Autodesk Fusion 360 part; units mm, degrees
note: some values were not read from the file. Set by a fixed rule: which sketch regions a step uses.
(part 2 of 2)
component "Component'''''''''''''" placed x (1, 0, 0) y (0, 1, 0) z (0, 0, 1) at (0, 0, 0)
component "Component''''''''''''''" placed x (1, 0, 0) y (0, 1, 0) z (0, 0, 1) at (0, 0, 0)
component "Component'''''''''''''''" placed x (1, 0, 0) y (0, 1, 0) z (0, 0, 1) at (0, 0, 0)
component "Component''''''''''''''''" placed x (1, 0, 0) y (0, 1, 0) z (0, 0, 1) at (0, 0, 0)
component "Component'''''''''''''''''" placed x (1, 0, 0) y (0, 1, 0) z (0, 0, 1) at (0, 0, 0)
component "Component''''''''''''''''''" placed x (1, 0, 0) y (0, 1, 0) z (0, 0, 1) at (0, 0, 0)
component "Component'''''''''''''''''''" placed x (1, 0, 0) y (0, 1, 0) z (0, 0, 1) at (0, 0, 0)
component "Component''''''''''''''''''''" placed x (1, 0, 0) y (0, 1, 0) z (0, 0, 1) at (0, 0, 0)
component "Component'''''''''''''''''''''" placed x (1, 0, 0) y (0, 1, 0) z (0, 0, 1) at (0, 0, 0)
component "Component''''''''''''''''''''''" placed x (1, 0, 0) y (0, 1, 0) z (0, 0, 1) at (0, 0, 0)
component "Component'''''''''''''''''''''''" placed x (1, 0, 0) y (0, 1, 0) z (0, 0, 1) at (0, 0, 0)
component "Component''''''''''''''''''''''''" placed x (1, 0, 0) y (0, 1, 0) z (0, 0, 1) at (0, 0, 0)
component "Component'''''''''''''''''''''''''" placed x (1, 0, 0) y (0, 1, 0) z (0, 0, 1) at (0, 0, 0)
component "Component''''''''''''''''''''''''''" placed x (1, 0, 0) y (0, 1, 0) z (0, 0, 1) at (0, 0, 0)
component "Component'''''''''''''''''''''''''''" placed x (1, 0, 0) y (0, 1, 0) z (0, 0, 1) at (0, 0, 0)
component "Component''''''''''''''''''''''''''''" placed x (1, 0, 0) y (0, 1, 0) z (0, 0, 1) at (0, 0, 0)
component "Component'''''''''''''''''''''''''''''" placed x (1, 0, 0) y (0, 1, 0) z (0, 0, 1) at (0, 0, 0)
component "Component''''''''''''''''''''''''''''''" placed x (1, 0, 0) y (0, 1, 0) z (0, 0, 1) at (0, 0, 0)
component "Component'''''''''''''''''''''''''''''''" placed x (1, 0, 0) y (0, 1, 0) z (0, 0, 1) at (0, 0, 0)
component "Component''''''''''''''''''''''''''''''''" placed x (1, 0, 0) y (0, 1, 0) z (0, 0, 1) at (0, 0, 0)
component "Component'''''''''''''''''''''''''''''''''" placed x (1, 0, 0) y (0, 1, 0) z (0, 0, 1) at (0, 0, 0)
component "Component''''''''''''''''''''''''''''''''''" placed x (1, 0, 0) y (0, 1, 0) z (0, 0, 1) at (0, 0, 0)
component "Component'''''''''''''''''''''''''''''''''''" placed x (1, 0, 0) y (0, 1, 0) z (0, 0, 1) at (0, 0, 0)
component "Component''''''''''''''''''''''''''''''''''''" placed x (1, 0, 0) y (0, 1, 0) z (0, 0, 1) at (0, 0, 0)
equation "FramingWidth = 105 in"
equation "FramingHeight = 99 in"
equation "d3 = FramingWidth"
equation "d4 = FramingHeight"
equation "d5 = FramingHeight"
equation "FlooringThickness = ( 3 / 4 ) * 1 in"
equation "DrywallThickness = ( 9 / 16 ) * 1 in"
equation "d8 = -DrywallThickness"
equation "d9 = FlooringThickness"
equation "DoorWidth = DoubleDoorWidth / 2" comment "From Center"
equation "d13 = ( -1 / 2 ) * 1 in"
equation "d14 = ( 1 / 2 ) * 1 in"
equation "PlasmaCutWidth = 1.25 in"
equation "d50 = DoorWidth"
equation "d51 = ( 1 / 2 ) * 1 in"
equation "d52 = DoorWidth"
equation "d56 = PlasmaCutWidth"
equation "d57 = PlasmaCutWidth"
equation "d58 = PlasmaCutWidth"
equation "DoubleDoorWidth = 62 in"
equation "FinalOpening = FramingWidth - Sheetrock * 2" comment "This is assuming sheetrock"
equation "Sheetrock = ( 9 / 16 ) * 1 in"
equation "PlasmaCutThickness = ( 3 / 16 ) * 1 in"
equation "SidelightSetback = 1.0625 in"
equation "d96 = SidelightSetback"
equation "d97 = PlasmaCutThickness"
equation "DoorCutSetback = ( 5 / 16 ) * 1 in"
equation "d105 = DoorCutSetback"
equation "d106 = PlasmaCutThickness"
equation "d113 = PlasmaCutWidth"
equation "d115 = PlasmaCutWidth"
equation "d116 = PlasmaCutWidth"
equation "d120 = ( 5 / 16 ) * 1 in"
equation "d121 = ( 5 / 16 ) * 1 in"
equation "d122 = PlasmaCutThickness"
equation "PanelSpacing = ( FramingHeight - 9.5625 in ) / 4"
equation "d130 = PanelSpacing"
equation "d131 = PanelSpacing"
equation "d132 = PanelSpacing"
equation "GlassThickness = 0.25 in"
equation "d150 = GlassThickness"
equation "HorizontalGlassOffset = ( 5 / 8 ) * 1 in"
equation "VerticalGlassOffset = ( 5 / 16 ) * 1 in"
equation "d170 = GlassThickness"
equation "d179 = ( 5 / 8 ) * 1 in"
equation "DoorHandleHole = 2.25 in"
equation "d219 = PlasmaCutThickness"
